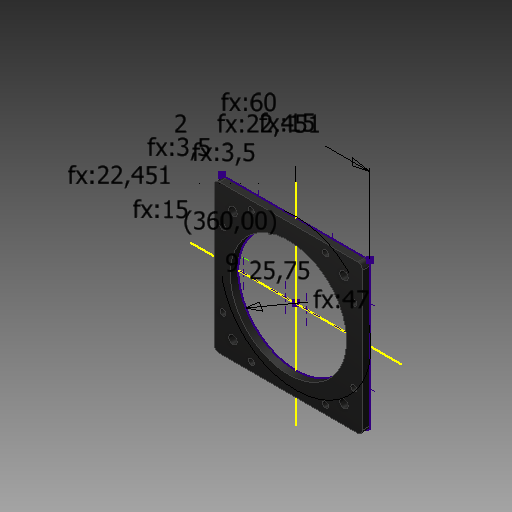
# Autodesk Inventor part: filler_ring-03
Saved by Autodesk Inventor 2019 (Build 230136000, 136)
## iProperties
Created: 2018-04-27
Part Number: filler_ring-03
Material: ABS Plastic
Document SubType Name: Modeling
Designer: Fierl
Density: 1.06 g/cm^3
Appearance: Smooth - White
Mass: 7.58584 g
Surface Area: 55.2729 cm^2
Volume: 7.15646 cm^3
Author: Fierl
Autodesk Inventor part; units mm, degrees
ref_plane "YZ Plane" through (0, 0, 0) normal (1, 0, 0) x (0, 1, 0)
ref_plane "XZ Plane" through (0, 0, 0) normal (0, 1, 0) x (-1, 0, 0)
ref_plane "XY Plane" through (0, 0, 0) normal (0, 0, 1) x (1, 0, 0)
sketch "Sketch1" plane through (0, 0, 0) normal (0, 0, 1) x (1, 0, 0)
  line L0 (0, -42.5799) -> (0, 42.5799) projected
  line L1 (-42.5799, 0) -> (42.5799, 0) projected
  line L2 (-28, 30) -> (28, 30)
  line L3 (30, 28) -> (30, -28)
  line L4 (28, -30) -> (-28, -30)
  line L5 (-30, -28) -> (-30, 28)
  arc A0 (-28, 30) -> (-30, 28) centre (-28, 28) ccw
  arc A1 (30, 28) -> (28, 30) centre (28, 28) ccw
  arc A2 (28, -30) -> (30, -28) centre (28, -28) ccw
  arc A3 (-30, -28) -> (-28, -30) centre (-28, -28) ccw
  circle A4 centre (0, 0) radius 23.5
  point P0 (-30, 30)
  point P1 (30, 30)
  point P2 (-22.4506, 22.4506)
  point P3 (-26.5, 15)
  point P4 (-15, 26.5)
  point P5 (-15, -26.5)
  point P6 (-22.4506, -22.4506)
  point P7 (-26.5, -15)
  point P8 (26.5, -15)
  point P9 (22.4506, -22.4506)
  point P10 (15, -26.5)
  point P11 (15, 26.5)
  point P12 (22.4506, 22.4506)
  point P13 (26.5, 15)
  point P14 (-21, 0)
  point P15 (21, 0)
  point P16 (-4.25, 0)
  point P17 (4.25, 0)
  point P18 (-24.6219, 5.3878)
  dimension "d0" = 60
  dimension "d1" = 2
  dimension "d2" = 22.4506
  dimension "d3" = 22.4506
  dimension "d4" = 15
  dimension "d5" = 15
  dimension "d6" = 3.5
  dimension "d7" = 3.5
  dimension "d10" = 360
  dimension "d28" = 9
  dimension "d36" = 25.75
  dimension "d48" = 47
  constraints: 8 end point, 8 point on circle, 8 tangent, 7 point on line, 5 centre point, 3 equal radius, 2 parallel, 2 perpendicular, 2 symmetric about line, 1 coincident, 1 horizontal, 15 other
  measures "d0" distance of point (-30, 30) point (30, 30)
  measures "d1" radius of A0
  measures "d2" distance from line of L0 point (-22.451, 22.451)
  measures "d3" distance from line of L1 point (-22.451, 22.451)
  measures "d4" distance from line of L1 point (-26.5, 15)
  measures "d5" distance from line of L0 point (-15, 26.5)
  measures "d6" distance from line of L2 point (-15, 26.5)
  measures "d7" distance from line of L5 point (-26.5, 15)
  measures "d28" distance from line of L5 point (-21, 0)
  measures "d36" distance from line of L5 point (-4.25, 0)
  measures "d48" diameter of A4
extrude "Extrusion2" add sketch "Sketch1" along normal blind 3 contours L4 A3 L5 L1 A4 L0 | L0 A4 L1 L3 A2 L4 | L1 L5 A0 L2 L0 A4 | A4 L0 L2 A1 L3 L1
hole "Hole5" at (15, -26.5, 0) at (26.5, -15, 0) at (-15, -26.5, 0) at (-26.5, -15, 0) at (-26.5, 15, 0) at (-15, 26.5, 0) at (15, 26.5, 0) at (26.5, 15, 0) direction (0, 0, 1) diameter 2.4 end through all clearance for "Countersunk Flat Head Screw DIN EN ISO 2009" size "M2" standard "DIN"
hole "Hole6" at (-22.4506, 22.4506, 0) at (-22.4506, -22.4506, 0) at (22.4506, -22.4506, 0) at (22.4506, 22.4506, 0) direction (0, 0, 1) diameter 3.4 end through all clearance for "Countersunk Flat Head Screw DIN EN ISO 2009" size "M3" standard "DIN"
equation "\"d0\" = backplate_width"
equation "\"d2\" = hole_distance"
equation "\"d3\" = hole_distance"
equation "\"d4\" = screw_distance_center"
equation "\"d5\" = screw_distance_center"
equation "\"d6\" = screw_distance_outside"
equation "\"d7\" = screw_distance_outside"
equation "\"d48\" = circle_dimension_inner"
equation "\"encoder_axis\" = 8"
equation "\"encoder_emboss\" = 0"
equation "\"encoders\" = 0"
equation "\"encoder_width\" = 27"
equation "\"front_plate_thickness\" = 2"
equation "\"glass_thickness\" = 2"
equation "\"screw_distance_outside\" = 3.5"
equation "\"encoder_rad\" = 49"
equation "\"encoder_extrude_hight\" = 3"
equation "\"screw_distance_center\" = 15"
equation "\"ring_top_thickness\" = 2"
equation "\"ring_outer_bevel_depth\" = 0.5"
equation "\"ring_depth\" = 6"
equation "\"ring_outer_bevel_height\" = 3"
equation "\"ring_inner_bevel_depth\" = 3.5"
equation "\"ring_thickness\" = 9"
equation "\"hole_from_center\" = 63.5"
equation "\"circle_dimension_inner\" = 47"
equation "\"circle_dimension\" = 56"
equation "\"backplate_width\" = 60"
equation "\"hole_distance\" = 22.45064"
body "Solid1"
